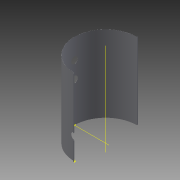
# Autodesk Inventor part: Upper Front Half New
Saved by Autodesk Inventor 2015 (Build 190159000, 159)
## iProperties
Created: 2014-07-11
Part Number: Upper Front Half New
Material: Generic
Document SubType Name: Modeling
Designer: I Rabey
Density: 1 g/cm^3
Appearance: Default
Author: I Rabey
Autodesk Inventor part; units mm, degrees
ref_plane "YZ Plane" through (0, 0, 0) normal (1, 0, 0) x (0, 1, 0)
sketch "Sketch1" plane through (0, 0, 0) normal (0, 1, 0) x (-1, 0, 0)
  arc A0 (0, -401) -> (0, 401) centre (0, 0) ccw
  line L0 (0, 0) -> (0, 401) construction
  line L1 (0, 0) -> (0, -401) construction
  arc A1 (0, -400) -> (0, 400) centre (0, 0) ccw
  line L2 (0, 0) -> (0, 400) construction
  line L3 (0, 0) -> (0, -400) construction
  line L4 (0, 400) -> (0, 401)
  line L5 (0, -401) -> (0, -400)
  dimension "d0" = 401
  dimension "d1" = 180
  dimension "d2" = 400
  dimension "d3" = 180
  constraints: 12 end point, 4 point on circle, 2 centre point, 2 coincident, 1 collinear, 1 point on line
  measures "d0" radius of A0
  measures "d1" angle of L0 L1
  measures "d2" radius of A1
  measures "d3" angle of L2 L3
extrude "Extrusion1" add sketch "Sketch1" along normal blind 980
sketch "Sketch2" plane through (0, 0, 0) normal (0, 1, 0) x (-1, 0, 0)
  line L0 (0, 400) -> (1, 400)
  line L1 (1, 400) -> (1, 416)
  line L2 (1, 416) -> (0, 416)
  line L3 (0, 416) -> (0, 400)
  line L4 (0, -400) -> (1, -400)
  line L5 (1, -400) -> (1, -416)
  line L6 (1, -416) -> (0, -416)
  line L7 (0, -416) -> (0, -400)
  point P0 (0, 0)
  dimension "d6" = 1
  dimension "d7" = 16
  dimension "d8" = 1
  dimension "d9" = 16
  constraints: 16 end point, 4 parallel, 2 horizontal, 2 perpendicular
  measures "d6" distance of L2.end L1.end
  measures "d7" distance of L0.end L1.end
  measures "d8" distance of L5.end L6.end
  measures "d9" distance of L4.end L5.end
extrude "Extrusion2" add sketch "Sketch2" along normal blind 980
ref_plane "Work Plane1" through (-401, 0, 0) normal (-1, 0, 0) x (0, -1, 0)
sketch "Sketch3" plane through (-401, 0, 0) normal (-1, 0, 0) x (0, -1, 0)
  circle A0 centre (-505.5, 0) radius 42
  line L0 (0, 400.9988) -> (0, -400.9988) projected
  point P0 (0, 0)
  dimension "d12" = 84
  dimension "d13" = 505.5
  constraints: 1 centre point
  measures "d12" diameter of A0
  measures "d13" distance from line of L0 A0.centre
sketch "Sketch4" plane through (-401, 0, 0) normal (-1, 0, 0) x (0, -1, 0)
  circle A0 centre (-720.5, 0) radius 42
  line L0 (0, 400.9988) -> (0, -400.9988) projected
  point P0 (0, 0)
  dimension "d14" = 84
  dimension "d15" = 720.5
  constraints: 1 centre point
  measures "d14" diameter of A0
  measures "d15" distance from line of L0 A0.centre
hole "Hole1" at (-401, 720.5, 0) direction (1, 0, 0) diameter 84 end through all
hole "Hole2" at (-401, 505.5, 0) direction (1, 0, 0) diameter 84 end through all
ref_plane "Work Plane2" through (0, 0, 408) normal (0, 0, 1) x (1, 0, 0)
sketch "Sketch5" plane through (0, 0, 408) normal (0, 0, 1) x (1, 0, 0)
  circle A0 centre (0, 277) radius 42
  line L0 (-1, 0) -> (-401, 0) projected
  point P0 (0, 0)
  dimension "d30" = 84
  dimension "d31" = 277
  constraints: 1 centre point
  measures "d30" diameter of A0
  measures "d31" distance from line of L0 A0.centre
extrude "Extrusion3" cut sketch "Sketch5" along normal blind 25 and the other way blind 25
body "Solid1"
